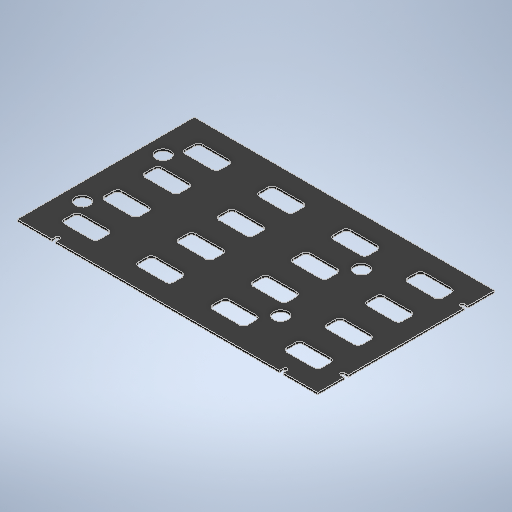
# Autodesk Inventor part: gasket V1
Saved by Autodesk Inventor 2025 (Build 290162000, 162)
## iProperties
Created: 2024-08-21
Part Number: gasket V1
Material: Rubber
Document SubType Name: Modeling
Designer: Caleb Fangmeier
Density: 0.93 g/cm^3
Appearance: Rubber - Black
Author: Caleb Fangmeier
Autodesk Inventor part; units mm, degrees
ref_plane "YZ Plane" through (0, 0, 0) normal (1, 0, 0) x (0, 1, 0)
ref_plane "XZ Plane" through (0, 0, 0) normal (0, 1, 0) x (-1, 0, 0)
ref_plane "XY Plane" through (0, 0, 0) normal (0, 0, 1) x (1, 0, 0)
sketch "Sketch1" plane through (0, 0, 0) normal (0, 1, 0) x (-1, 0, 0)
  arc A0 (-42.3717, -8.6221) -> (-45.3717, -11.6221) centre (-42.3717, -11.6221) ccw
  line L0 (-42.3717, -8.6221) -> (-21.3717, -8.6221)
  arc A1 (-18.3717, -11.6221) -> (-21.3717, -8.6221) centre (-21.3717, -11.6221) ccw
  line L1 (-18.3717, -11.6221) -> (-18.3717, -18.6221)
  arc A2 (-21.3717, -21.6221) -> (-18.3717, -18.6221) centre (-21.3717, -18.6221) ccw
  line L2 (-21.3717, -21.6221) -> (-42.3717, -21.6221)
  arc A3 (-45.3717, -18.6221) -> (-42.3717, -21.6221) centre (-42.3717, -18.6221) ccw
  line L3 (-45.3717, -18.6221) -> (-45.3717, -11.6221)
  arc A4 (71.6283, -8.6221) -> (68.6283, -11.6221) centre (71.6283, -11.6221) ccw
  line L4 (71.6283, -8.6221) -> (92.6283, -8.6221)
  arc A5 (95.6283, -11.6221) -> (92.6283, -8.6221) centre (92.6283, -11.6221) ccw
  line L5 (95.6283, -11.6221) -> (95.6283, -18.6221)
  arc A6 (92.6283, -21.6221) -> (95.6283, -18.6221) centre (92.6283, -18.6221) ccw
  line L6 (92.6283, -21.6221) -> (71.6283, -21.6221)
  arc A7 (68.6283, -18.6221) -> (71.6283, -21.6221) centre (71.6283, -18.6221) ccw
  line L7 (68.6283, -18.6221) -> (68.6283, -11.6221)
  arc A8 (14.6283, -39.6221) -> (11.6283, -42.6221) centre (14.6283, -42.6221) ccw
  line L8 (14.6283, -39.6221) -> (35.6283, -39.6221)
  arc A9 (38.6283, -42.6221) -> (35.6283, -39.6221) centre (35.6283, -42.6221) ccw
  line L9 (38.6283, -42.6221) -> (38.6283, -49.6221)
  arc A10 (35.6283, -52.6221) -> (38.6283, -49.6221) centre (35.6283, -49.6221) ccw
  line L10 (35.6283, -52.6221) -> (14.6283, -52.6221)
  arc A11 (11.6283, -49.6221) -> (14.6283, -52.6221) centre (14.6283, -49.6221) ccw
  line L11 (11.6283, -49.6221) -> (11.6283, -42.6221)
  arc A12 (14.6283, 53.3779) -> (11.6283, 50.3779) centre (14.6283, 50.3779) ccw
  line L12 (14.6283, 53.3779) -> (35.6283, 53.3779)
  arc A13 (38.6283, 50.3779) -> (35.6283, 53.3779) centre (35.6283, 50.3779) ccw
  line L13 (38.6283, 50.3779) -> (38.6283, 43.3779)
  arc A14 (35.6283, 40.3779) -> (38.6283, 43.3779) centre (35.6283, 43.3779) ccw
  line L14 (35.6283, 40.3779) -> (14.6283, 40.3779)
  arc A15 (11.6283, 43.3779) -> (14.6283, 40.3779) centre (14.6283, 43.3779) ccw
  line L15 (11.6283, 43.3779) -> (11.6283, 50.3779)
  arc A16 (-42.3717, 53.3779) -> (-45.3717, 50.3779) centre (-42.3717, 50.3779) ccw
  line L16 (-42.3717, 53.3779) -> (-21.3717, 53.3779)
  arc A17 (-18.3717, 50.3779) -> (-21.3717, 53.3779) centre (-21.3717, 50.3779) ccw
  line L17 (-18.3717, 50.3779) -> (-18.3717, 43.3779)
  arc A18 (-21.3717, 40.3779) -> (-18.3717, 43.3779) centre (-21.3717, 43.3779) ccw
  line L18 (-21.3717, 40.3779) -> (-42.3717, 40.3779)
  arc A19 (-45.3717, 43.3779) -> (-42.3717, 40.3779) centre (-42.3717, 43.3779) ccw
  line L19 (-45.3717, 43.3779) -> (-45.3717, 50.3779)
  arc A20 (-42.3717, -39.6221) -> (-45.3717, -42.6221) centre (-42.3717, -42.6221) ccw
  line L20 (-42.3717, -39.6221) -> (-21.3717, -39.6221)
  arc A21 (-18.3717, -42.6221) -> (-21.3717, -39.6221) centre (-21.3717, -42.6221) ccw
  line L21 (-18.3717, -42.6221) -> (-18.3717, -49.6221)
  arc A22 (-21.3717, -52.6221) -> (-18.3717, -49.6221) centre (-21.3717, -49.6221) ccw
  line L22 (-21.3717, -52.6221) -> (-42.3717, -52.6221)
  arc A23 (-45.3717, -49.6221) -> (-42.3717, -52.6221) centre (-42.3717, -49.6221) ccw
  line L23 (-45.3717, -49.6221) -> (-45.3717, -42.6221)
  arc A24 (14.6283, -8.6221) -> (11.6283, -11.6221) centre (14.6283, -11.6221) ccw
  line L24 (14.6283, -8.6221) -> (35.6283, -8.6221)
  arc A25 (38.6283, -11.6221) -> (35.6283, -8.6221) centre (35.6283, -11.6221) ccw
  line L25 (38.6283, -11.6221) -> (38.6283, -18.6221)
  arc A26 (35.6283, -21.6221) -> (38.6283, -18.6221) centre (35.6283, -18.6221) ccw
  line L26 (35.6283, -21.6221) -> (14.6283, -21.6221)
  arc A27 (11.6283, -18.6221) -> (14.6283, -21.6221) centre (14.6283, -18.6221) ccw
  line L27 (11.6283, -18.6221) -> (11.6283, -11.6221)
  arc A28 (-99.3717, -8.6221) -> (-102.3717, -11.6221) centre (-99.3717, -11.6221) ccw
  line L28 (-99.3717, -8.6221) -> (-78.3717, -8.6221)
  arc A29 (-75.3717, -11.6221) -> (-78.3717, -8.6221) centre (-78.3717, -11.6221) ccw
  line L29 (-75.3717, -11.6221) -> (-75.3717, -18.6221)
  arc A30 (-78.3717, -21.6221) -> (-75.3717, -18.6221) centre (-78.3717, -18.6221) ccw
  line L30 (-78.3717, -21.6221) -> (-99.3717, -21.6221)
  arc A31 (-102.3717, -18.6221) -> (-99.3717, -21.6221) centre (-99.3717, -18.6221) ccw
  line L31 (-102.3717, -18.6221) -> (-102.3717, -11.6221)
  arc A32 (-42.3717, 22.3779) -> (-45.3717, 19.3779) centre (-42.3717, 19.3779) ccw
  line L32 (-42.3717, 22.3779) -> (-21.3717, 22.3779)
  arc A33 (-18.3717, 19.3779) -> (-21.3717, 22.3779) centre (-21.3717, 19.3779) ccw
  line L33 (-18.3717, 19.3779) -> (-18.3717, 12.3779)
  arc A34 (-21.3717, 9.3779) -> (-18.3717, 12.3779) centre (-21.3717, 12.3779) ccw
  line L34 (-21.3717, 9.3779) -> (-42.3717, 9.3779)
  arc A35 (-45.3717, 12.3779) -> (-42.3717, 9.3779) centre (-42.3717, 12.3779) ccw
  line L35 (-45.3717, 12.3779) -> (-45.3717, 19.3779)
  arc A36 (71.6283, 22.3779) -> (68.6283, 19.3779) centre (71.6283, 19.3779) ccw
  line L36 (71.6283, 22.3779) -> (92.6283, 22.3779)
  arc A37 (95.6283, 19.3779) -> (92.6283, 22.3779) centre (92.6283, 19.3779) ccw
  line L37 (95.6283, 19.3779) -> (95.6283, 12.3779)
  arc A38 (92.6283, 9.3779) -> (95.6283, 12.3779) centre (92.6283, 12.3779) ccw
  line L38 (92.6283, 9.3779) -> (71.6283, 9.3779)
  arc A39 (68.6283, 12.3779) -> (71.6283, 9.3779) centre (71.6283, 12.3779) ccw
  line L39 (68.6283, 12.3779) -> (68.6283, 19.3779)
  arc A40 (71.6283, -39.6221) -> (68.6283, -42.6221) centre (71.6283, -42.6221) ccw
  line L40 (71.6283, -39.6221) -> (92.6283, -39.6221)
  arc A41 (95.6283, -42.6221) -> (92.6283, -39.6221) centre (92.6283, -42.6221) ccw
  line L41 (95.6283, -42.6221) -> (95.6283, -49.6221)
  arc A42 (92.6283, -52.6221) -> (95.6283, -49.6221) centre (92.6283, -49.6221) ccw
  line L42 (92.6283, -52.6221) -> (71.6283, -52.6221)
  arc A43 (68.6283, -49.6221) -> (71.6283, -52.6221) centre (71.6283, -49.6221) ccw
  line L43 (68.6283, -49.6221) -> (68.6283, -42.6221)
  arc A44 (71.6283, 53.3779) -> (68.6283, 50.3779) centre (71.6283, 50.3779) ccw
  line L44 (71.6283, 53.3779) -> (92.6283, 53.3779)
  arc A45 (95.6283, 50.3779) -> (92.6283, 53.3779) centre (92.6283, 50.3779) ccw
  line L45 (95.6283, 50.3779) -> (95.6283, 43.3779)
  arc A46 (92.6283, 40.3779) -> (95.6283, 43.3779) centre (92.6283, 43.3779) ccw
  line L46 (92.6283, 40.3779) -> (71.6283, 40.3779)
  arc A47 (68.6283, 43.3779) -> (71.6283, 40.3779) centre (71.6283, 43.3779) ccw
  line L47 (68.6283, 43.3779) -> (68.6283, 50.3779)
  arc A48 (-78.3717, 40.3779) -> (-75.3717, 43.3779) centre (-78.3717, 43.3779) ccw
  line L48 (-78.3717, 40.3779) -> (-99.3717, 40.3779)
  arc A49 (-102.3717, 43.3779) -> (-99.3717, 40.3779) centre (-99.3717, 43.3779) ccw
  line L49 (-102.3717, 43.3779) -> (-102.3717, 50.3779)
  arc A50 (-99.3717, 53.3779) -> (-102.3717, 50.3779) centre (-99.3717, 50.3779) ccw
  line L50 (-99.3717, 53.3779) -> (-78.3717, 53.3779)
  arc A51 (-75.3717, 50.3779) -> (-78.3717, 53.3779) centre (-78.3717, 50.3779) ccw
  line L51 (-75.3717, 50.3779) -> (-75.3717, 43.3779)
  arc A52 (-99.3717, -39.6221) -> (-102.3717, -42.6221) centre (-99.3717, -42.6221) ccw
  line L52 (-99.3717, -39.6221) -> (-78.3717, -39.6221)
  arc A53 (-75.3717, -42.6221) -> (-78.3717, -39.6221) centre (-78.3717, -42.6221) ccw
  line L53 (-75.3717, -42.6221) -> (-75.3717, -49.6221)
  arc A54 (-78.3717, -52.6221) -> (-75.3717, -49.6221) centre (-78.3717, -49.6221) ccw
  line L54 (-78.3717, -52.6221) -> (-99.3717, -52.6221)
  arc A55 (-102.3717, -49.6221) -> (-99.3717, -52.6221) centre (-99.3717, -49.6221) ccw
  line L55 (-102.3717, -49.6221) -> (-102.3717, -42.6221)
  arc A56 (14.6283, 22.3779) -> (11.6283, 19.3779) centre (14.6283, 19.3779) ccw
  line L56 (14.6283, 22.3779) -> (35.6283, 22.3779)
  arc A57 (38.6283, 19.3779) -> (35.6283, 22.3779) centre (35.6283, 19.3779) ccw
  line L57 (38.6283, 19.3779) -> (38.6283, 12.3779)
  arc A58 (35.6283, 9.3779) -> (38.6283, 12.3779) centre (35.6283, 12.3779) ccw
  line L58 (35.6283, 9.3779) -> (14.6283, 9.3779)
  arc A59 (11.6283, 12.3779) -> (14.6283, 9.3779) centre (14.6283, 12.3779) ccw
  line L59 (11.6283, 12.3779) -> (11.6283, 19.3779)
  arc A60 (-99.3717, 22.3779) -> (-102.3717, 19.3779) centre (-99.3717, 19.3779) ccw
  line L60 (-99.3717, 22.3779) -> (-78.3717, 22.3779)
  arc A61 (-75.3717, 19.3779) -> (-78.3717, 22.3779) centre (-78.3717, 19.3779) ccw
  line L61 (-75.3717, 19.3779) -> (-75.3717, 12.3779)
  arc A62 (-78.3717, 9.3779) -> (-75.3717, 12.3779) centre (-78.3717, 12.3779) ccw
  line L62 (-78.3717, 9.3779) -> (-99.3717, 9.3779)
  arc A63 (-102.3717, 12.3779) -> (-99.3717, 9.3779) centre (-99.3717, 12.3779) ccw
  line L63 (-102.3717, 12.3779) -> (-102.3717, 19.3779)
  line L64 (113.6283, 68.3779) -> (-117.3717, 68.3779)
  line L65 (-117.3717, 68.3779) -> (-117.3717, -67.6221)
  line L66 (-117.3717, -67.6221) -> (113.6283, -67.6221)
  line L67 (113.6283, -67.6221) -> (113.6283, 68.3779)
  circle A64 centre (-51.8717, 31.3779) radius 5.5565
  circle A65 centre (100.5283, -30.6221) radius 5.5565
  circle A66 centre (-51.8717, -30.6221) radius 5.5565
  circle A67 centre (100.5283, 31.3779) radius 5.5565
  circle A68 centre (-89.3717, 65.3779) radius 1.5
  circle A69 centre (-114.3717, 46.3779) radius 1.5
  circle A70 centre (-114.3717, -45.6221) radius 1.5
  circle A71 centre (85.6283, 65.3779) radius 1.5
  point P0 (0, 0)
  point P1 (113.6283, -67.6221)
  point P2 (-75.3717, -11.6221)
  point P3 (-75.3717, 43.3779)
  point P4 (-21.3717, -52.6221)
  point P5 (35.6283, 9.3779)
  point P6 (95.6283, -42.6221)
  point P7 (71.6283, -52.6221)
  point P8 (71.6283, -39.6221)
  point P9 (38.6283, -18.6221)
  point P10 (71.6283, 9.3779)
  point P11 (-78.3717, 9.3779)
  point P12 (-99.3717, 9.3779)
  point P13 (-18.3717, 50.3779)
  point P14 (-45.3717, 50.3779)
  point P15 (-45.3717, 19.3779)
  point P16 (-18.3717, 12.3779)
  point P17 (-21.3717, 9.3779)
  point P18 (-42.3717, 9.3779)
  point P19 (14.6283, -39.6221)
  point P20 (-18.3717, -11.6221)
  point P21 (-21.3717, -21.6221)
  constraints: 136 end point, 128 point on circle, 72 centre point
extrude "Extrusion1" add sketch "Sketch1" along normal blind 1.5875
sketch "Sketch2" plane through (0, 1.5875, 0) normal (0, 1, 0) x (1, 0, 0)
  circle A0 centre (114.3717, 45.6221) radius 1.5 projected
  line L0 (117.3717, -68.3779) -> (117.3717, 67.6221) projected
  line L1 (114.3717, 44.1221) -> (117.3717, 44.1221)
  line L2 (117.3717, 44.1221) -> (117.3717, 47.1221)
  line L3 (117.3717, 47.1221) -> (114.3717, 47.1221)
  line L4 (114.3717, 47.1221) -> (114.3717, 44.1221)
  circle A1 centre (114.3717, -46.3779) radius 1.5 projected
  line L5 (114.3717, -47.8779) -> (117.3717, -47.8779)
  line L6 (117.3717, -47.8779) -> (117.3717, -44.8776)
  line L7 (117.3717, -44.8776) -> (114.3717, -44.8776)
  line L8 (114.3717, -44.8776) -> (114.3717, -47.8779)
  circle A2 centre (114.3717, -46.3779) radius 1.5 projected
  circle A3 centre (89.3717, -65.3779) radius 1.5 projected
  line L9 (-113.6283, -68.3779) -> (117.3717, -68.3779) projected
  line L10 (90.8717, -65.3779) -> (87.8717, -65.3779)
  line L11 (87.8717, -65.3779) -> (87.8717, -68.3779)
  line L12 (87.8717, -68.3779) -> (90.8717, -68.3779)
  line L13 (90.8717, -68.3779) -> (90.8717, -65.3779)
  circle A4 centre (-85.6283, -65.3779) radius 1.5 projected
  line L14 (-84.1283, -65.3779) -> (-87.1283, -65.3779)
  line L15 (-87.1283, -65.3779) -> (-87.1283, -68.3779)
  line L16 (-87.1283, -68.3779) -> (-84.1283, -68.3779)
  line L17 (-84.1283, -68.3779) -> (-84.1283, -65.3779)
  point P0 (0, 0)
  point P1 (114.3717, -44.8779)
  dimension "d2" = 3.0003
  dimension "d3" = 3
  dimension "d4" = 3
  dimension "d5" = 3
  constraints: 32 end point, 8 parallel, 5 point on line, 4 horizontal, 4 perpendicular, 2 horizontal alignment, 2 vertical alignment, 9 other
  measures "d2" distance of L7.end L5.start
  measures "d3" distance of L3.end L1.start
  measures "d4" distance of L10.start L10.end
  measures "d5" distance of L14.start L14.end
extrude "Extrusion2" cut sketch "Sketch2" against normal through all contours A0 L3 L0 L1 | L9 L15 A4 L17 | L9 L11 A3 L13 | L0 L5 A1 L7
body "Solid1"
